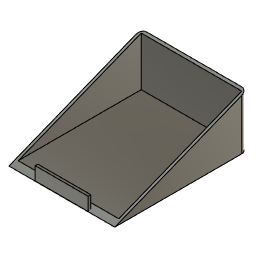
PhoneHolder v1 (Autodesk Fusion 360 design; units mm, degrees)
Autodesk Fusion 360 part; units mm, degrees
sketch "Sketch1" plane through (0, 0, 0) normal (0, 0, 1) x (1, 0, 0)
  line L0 (0, 0) -> (52.7547, 0)
  line L1 (52.7547, 0) -> (52.7547, 76.2575)
  line L2 (52.7547, 76.2575) -> (0, 76.2575)
  line L3 (0, 76.2575) -> (0, 0)
  constraint horizontal L0
  constraint vertical L1
  constraint horizontal L2
  constraint vertical L3
  constraint coincident L0.start L3.end
sketch "Sketch2" plane through (0, 0, 0) normal (0, 0, 1) x (1, 0, 0)
  line L0 (0, 0) -> (38.1, 0)
  line L1 (38.1, 0) -> (38.1, 63.5)
  line L2 (38.1, 63.5) -> (0, 63.5)
  line L3 (0, 63.5) -> (0, 0)
  dimension "d6" = 38.1
  dimension "d7" = 63.5
  constraint horizontal L0
  constraint vertical L1
  constraint horizontal L2
  constraint vertical L3
  constraint coincident L0.start L3.end
  measures "d6" distance of L0.start L0.end
  measures "d7" distance of L0.start L2.end
sketch "Sketch3" plane through (0, 0, 0) normal (1, 0, 0) x (0, 1, 0)
  line L0 (0, 0) -> (63.5027, 25.2897)
  line L1 (63.5027, 25.2897) -> (63.5027, 0)
  line L2 (63.5027, 0) -> (0, 0)
  constraint coincident L0.start L2.end
  constraint vertical L1
  constraint perpendicular L1 L2
extrude "Extrude3" add sketch "Sketch3" along normal blind 50.8 makes body 1
shell "Shell3" thickness 1.27 removed faces 1 at (16.9333, 21.1676, 8.4299) on bodies 1
fillet "Fillet2" radius 2.54 2 edges at (50.8, 63.5027, 12.6449) (0, 63.5027, 12.6449) on bodies 1
sketch "Sketch4" plane through (0, 0, 0) normal (0, 0, 1) x (1, 0, 0)
  line L0 (12.483, 0.1021) -> (37.883, 0.1021)
  line L1 (37.883, 0.1021) -> (37.883, 1.3721)
  line L2 (37.883, 1.3721) -> (12.483, 1.3721)
  line L3 (12.483, 1.3721) -> (12.483, 0.1021)
  dimension "d16" = 25.4
  dimension "d17" = 1.27
  constraint horizontal L0
  constraint vertical L1
  constraint horizontal L2
  constraint vertical L3
  measures "d16" distance of L0.start L0.end
  measures "d17" distance of L0.start L2.end
extrude "Extrude4" add sketch "Sketch4" along normal blind 6.35 separate body makes body 2
